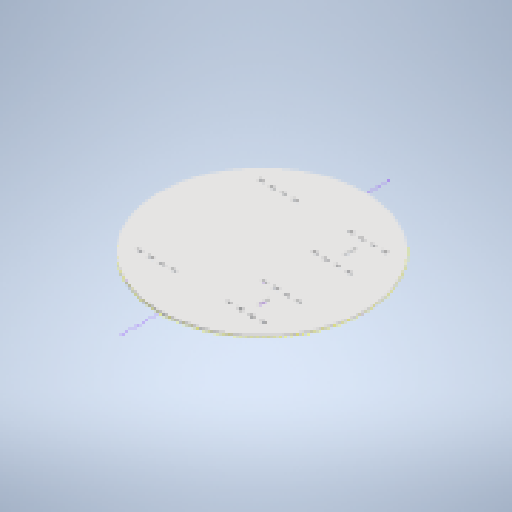
# Autodesk Inventor part: Osn. platform
Saved by Autodesk Inventor 2023.1 (Build 271208000, 208)
## iProperties
Created: 2023-03-13
Part Number: Osn. platform
Material: Типовые
Document SubType Name: Modeling
Designer: User
Density: 1 g/cm^3
Appearance: По умолчанию
Author: User
Autodesk Inventor part; units mm, degrees
ref_plane "YZ Plane" through (0, 0, 0) normal (1, 0, 0) x (0, 1, 0)
ref_plane "XZ Plane" through (0, 0, 0) normal (0, 1, 0) x (-1, 0, 0)
ref_plane "XY Plane" through (0, 0, 0) normal (0, 0, 1) x (1, 0, 0)
sketch "Основ. платформа" plane through (0, 0, 0) normal (0, 1, 0) x (-1, 0, 0)
  circle A0 centre (0, 0) radius 240
  dimension "d117" = 480
  constraints: 1 centre point, 1 coincident
  measures "d117" diameter of A0
extrude "Осн. платформа" add sketch "Основ. платформа" along normal blind 5
sketch "Эскиз14" plane through (0, 5, 0) normal (0, 1, 0) x (1, 0, 0)
  line L0 (137.6204, -61.9298) -> (150.9061, -61.9298) projected
  line L1 (150.9061, -61.9298) -> (150.9061, -55.9298) projected
  line L2 (137.6204, -55.9298) -> (150.9061, -55.9298) projected
  line L3 (137.6204, -61.9298) -> (137.6204, -55.9298) projected
  line L4 (111.049, -61.9298) -> (124.3347, -61.9298) projected
  line L5 (124.3347, -61.9298) -> (124.3347, -55.9298) projected
  line L6 (111.049, -55.9298) -> (124.3347, -55.9298) projected
  line L7 (111.049, -61.9298) -> (111.049, -55.9298) projected
  line L8 (84.4776, -61.9298) -> (97.7633, -61.9298) projected
  line L9 (97.7633, -61.9298) -> (97.7633, -55.9298) projected
  line L10 (84.4776, -55.9298) -> (97.7633, -55.9298) projected
  line L11 (84.4776, -61.9298) -> (84.4776, -55.9298) projected
  line L12 (57.9061, -144.9298) -> (71.1919, -144.9298) projected
  line L13 (71.1919, -144.9298) -> (71.1919, -138.9298) projected
  line L14 (57.9061, -138.9298) -> (71.1919, -138.9298) projected
  line L15 (57.9061, -144.9298) -> (57.9061, -138.9298) projected
  line L16 (84.4776, -144.9298) -> (97.7633, -144.9298) projected
  line L17 (97.7633, -144.9298) -> (97.7633, -138.9298) projected
  line L18 (84.4776, -138.9298) -> (97.7633, -138.9298) projected
  line L19 (84.4776, -144.9298) -> (84.4776, -138.9298) projected
  line L20 (111.049, -144.9298) -> (124.3347, -144.9298) projected
  line L21 (124.3347, -144.9298) -> (124.3347, -138.9298) projected
  line L22 (111.049, -138.9298) -> (124.3347, -138.9298) projected
  line L23 (111.049, -144.9298) -> (111.049, -138.9298) projected
  line L24 (137.6204, -144.9298) -> (150.9061, -144.9298) projected
  line L25 (150.9061, -144.9298) -> (150.9061, -138.9298) projected
  line L26 (137.6204, -138.9298) -> (150.9061, -138.9298) projected
  line L27 (137.6204, -144.9298) -> (137.6204, -138.9298) projected
  line L28 (101.4061, -87.5965) -> (101.4061, -113.2631) projected
  line L29 (101.4061, -113.2631) -> (107.4061, -113.2631) projected
  line L30 (107.4061, -113.2631) -> (107.4061, -87.5965) projected
  line L31 (107.4061, -87.5965) -> (101.4061, -87.5965) projected
  line L32 (57.9061, -61.9298) -> (71.1919, -61.9298) projected
  line L33 (71.1919, -61.9298) -> (71.1919, -55.9298) projected
  line L34 (57.9061, -55.9298) -> (71.1919, -55.9298) projected
  line L35 (57.9061, -61.9298) -> (57.9061, -55.9298) projected
  line L36 (-295.6598, 0) -> (443.256, 0) construction
  line L37 (0, -368.1913) -> (0, 462.3459) construction
  line L38 (-58.1024, -138.9298) -> (-70.9595, -138.9298) projected
  line L39 (-70.9595, -138.9298) -> (-70.9595, -144.9298) projected
  line L40 (-58.1024, -144.9298) -> (-70.9595, -144.9298) projected
  line L41 (-58.1024, -138.9298) -> (-58.1024, -144.9298) projected
  line L42 (-83.8167, -138.9298) -> (-96.6738, -138.9298) projected
  line L43 (-96.6738, -138.9298) -> (-96.6738, -144.9298) projected
  line L44 (-83.8167, -144.9298) -> (-96.6738, -144.9298) projected
  line L45 (-83.8167, -138.9298) -> (-83.8167, -144.9298) projected
  line L46 (-109.531, -138.9298) -> (-122.3881, -138.9298) projected
  line L47 (-122.3881, -138.9298) -> (-122.3881, -144.9298) projected
  line L48 (-109.531, -144.9298) -> (-122.3881, -144.9298) projected
  line L49 (-109.531, -138.9298) -> (-109.531, -144.9298) projected
  line L50 (-135.2452, -138.9298) -> (-148.1024, -138.9298) projected
  line L51 (-148.1024, -138.9298) -> (-148.1024, -144.9298) projected
  line L52 (-135.2452, -144.9298) -> (-148.1024, -144.9298) projected
  line L53 (-135.2452, -138.9298) -> (-135.2452, -144.9298) projected
  line L54 (-58.1024, -144.9298) -> (-148.1024, -144.9298) construction
  line L55 (-148.1024, -144.9298) -> (-148.1024, -100.7298) construction
  line L56 (-148.1024, -100.7298) -> (-58.1024, -100.7298) construction
  line L57 (-58.1024, -100.7298) -> (-58.1024, -144.9298) construction
  line L58 (-58.1024, -122.8298) -> (-148.1024, -122.8298) construction
  line L59 (137.6204, -138.9298) -> (124.3347, -144.9298) construction
  circle A0 centre (130.9776, -141.9298) radius 1.5
  circle A1 centre (104.2556, -141.9298) radius 1.5
  circle A2 centre (77.5336, -141.9298) radius 1.5
  circle A3 centre (130.9776, -58.9298) radius 1.5
  circle A4 centre (104.2556, -58.9298) radius 1.5
  circle A5 centre (77.5336, -58.9298) radius 1.5
  line L60 (-70.9595, -138.9298) -> (-83.8167, -144.9298) construction
  circle A6 centre (-77.3881, -141.9298) radius 1.5
  circle A7 centre (-103.2571, -141.9298) radius 1.5
  circle A8 centre (-129.1261, -141.9298) radius 1.5
  line L61 (-58.1024, -106.7298) -> (-70.9595, -106.7298)
  line L62 (-70.9595, -106.7298) -> (-70.9595, -100.7298)
  line L63 (-58.1024, -100.7298) -> (-70.9595, -100.7298)
  line L64 (-58.1024, -106.7298) -> (-58.1024, -100.7298)
  line L65 (-83.8167, -106.7298) -> (-96.6738, -106.7298)
  line L66 (-96.6738, -106.7298) -> (-96.6738, -100.7298)
  line L67 (-83.8167, -100.7298) -> (-96.6738, -100.7298)
  line L68 (-83.8167, -106.7298) -> (-83.8167, -100.7298)
  line L69 (-109.531, -106.7298) -> (-122.3881, -106.7298)
  line L70 (-122.3881, -106.7298) -> (-122.3881, -100.7298)
  line L71 (-109.531, -100.7298) -> (-122.3881, -100.7298)
  line L72 (-109.531, -106.7298) -> (-109.531, -100.7298)
  line L73 (-135.2452, -106.7298) -> (-148.1024, -106.7298)
  line L74 (-148.1024, -106.7298) -> (-148.1024, -100.7298)
  line L75 (-135.2452, -100.7298) -> (-148.1024, -100.7298)
  line L76 (-135.2452, -106.7298) -> (-135.2452, -100.7298)
  circle A9 centre (-77.3881, -103.7298) radius 1.5
  circle A10 centre (-103.2571, -103.7298) radius 1.5
  circle A11 centre (-129.1261, -103.7298) radius 1.5
  line L77 (137.6204, 61.9298) -> (150.9061, 61.9298)
  line L78 (150.9061, 61.9298) -> (150.9061, 55.9298)
  line L79 (137.6204, 55.9298) -> (150.9061, 55.9298)
  line L80 (137.6204, 61.9298) -> (137.6204, 55.9298)
  line L81 (111.049, 61.9298) -> (124.3347, 61.9298)
  line L82 (124.3347, 61.9298) -> (124.3347, 55.9298)
  line L83 (111.049, 55.9298) -> (124.3347, 55.9298)
  line L84 (111.049, 61.9298) -> (111.049, 55.9298)
  line L85 (84.4776, 61.9298) -> (97.7633, 61.9298)
  line L86 (97.7633, 61.9298) -> (97.7633, 55.9298)
  line L87 (84.4776, 55.9298) -> (97.7633, 55.9298)
  line L88 (84.4776, 61.9298) -> (84.4776, 55.9298)
  line L89 (57.9061, 144.9298) -> (71.1919, 144.9298)
  line L90 (71.1919, 144.9298) -> (71.1919, 138.9298)
  line L91 (57.9061, 138.9298) -> (71.1919, 138.9298)
  line L92 (57.9061, 144.9298) -> (57.9061, 138.9298)
  line L93 (84.4776, 144.9298) -> (97.7633, 144.9298)
  line L94 (97.7633, 144.9298) -> (97.7633, 138.9298)
  line L95 (84.4776, 138.9298) -> (97.7633, 138.9298)
  line L96 (84.4776, 144.9298) -> (84.4776, 138.9298)
  line L97 (111.049, 144.9298) -> (124.3347, 144.9298)
  line L98 (124.3347, 144.9298) -> (124.3347, 138.9298)
  line L99 (111.049, 138.9298) -> (124.3347, 138.9298)
  line L100 (111.049, 144.9298) -> (111.049, 138.9298)
  line L101 (137.6204, 144.9298) -> (150.9061, 144.9298)
  line L102 (150.9061, 144.9298) -> (150.9061, 138.9298)
  line L103 (137.6204, 138.9298) -> (150.9061, 138.9298)
  line L104 (137.6204, 144.9298) -> (137.6204, 138.9298)
  line L105 (101.4061, 87.5965) -> (101.4061, 113.2631)
  line L106 (101.4061, 113.2631) -> (107.4061, 113.2631)
  line L107 (107.4061, 113.2631) -> (107.4061, 87.5965)
  line L108 (107.4061, 87.5965) -> (101.4061, 87.5965)
  line L109 (57.9061, 61.9298) -> (71.1919, 61.9298)
  line L110 (71.1919, 61.9298) -> (71.1919, 55.9298)
  line L111 (57.9061, 55.9298) -> (71.1919, 55.9298)
  line L112 (57.9061, 61.9298) -> (57.9061, 55.9298)
  line L113 (0, 368.1913) -> (0, -462.3459) construction
  line L114 (-58.1024, 138.9298) -> (-70.9595, 138.9298)
  line L115 (-70.9595, 138.9298) -> (-70.9595, 144.9298)
  line L116 (-58.1024, 144.9298) -> (-70.9595, 144.9298)
  line L117 (-58.1024, 138.9298) -> (-58.1024, 144.9298)
  line L118 (-83.8167, 138.9298) -> (-96.6738, 138.9298)
  line L119 (-96.6738, 138.9298) -> (-96.6738, 144.9298)
  line L120 (-83.8167, 144.9298) -> (-96.6738, 144.9298)
  line L121 (-83.8167, 138.9298) -> (-83.8167, 144.9298)
  line L122 (-109.531, 138.9298) -> (-122.3881, 138.9298)
  line L123 (-122.3881, 138.9298) -> (-122.3881, 144.9298)
  line L124 (-109.531, 144.9298) -> (-122.3881, 144.9298)
  line L125 (-109.531, 138.9298) -> (-109.531, 144.9298)
  line L126 (-135.2452, 138.9298) -> (-148.1024, 138.9298)
  line L127 (-148.1024, 138.9298) -> (-148.1024, 144.9298)
  line L128 (-135.2452, 144.9298) -> (-148.1024, 144.9298)
  line L129 (-135.2452, 138.9298) -> (-135.2452, 144.9298)
  line L130 (-58.1024, 144.9298) -> (-148.1024, 144.9298) construction
  line L131 (-148.1024, 100.7298) -> (-58.1024, 100.7298) construction
  line L132 (137.6204, 138.9298) -> (124.3347, 144.9298) construction
  circle A12 centre (130.9776, 141.9298) radius 1.5
  circle A13 centre (104.2556, 141.9298) radius 1.5
  circle A14 centre (77.5336, 141.9298) radius 1.5
  circle A15 centre (130.9776, 58.9298) radius 1.5
  circle A16 centre (104.2556, 58.9298) radius 1.5
  circle A17 centre (77.5336, 58.9298) radius 1.5
  line L133 (-70.9595, 138.9298) -> (-83.8167, 144.9298) construction
  circle A18 centre (-77.3881, 141.9298) radius 1.5
  circle A19 centre (-103.2571, 141.9298) radius 1.5
  circle A20 centre (-129.1261, 141.9298) radius 1.5
  line L134 (-122.3881, 106.7298) -> (-122.3881, 100.7298)
  line L135 (-109.531, 100.7298) -> (-122.3881, 100.7298)
  line L136 (-109.531, 106.7298) -> (-109.531, 100.7298)
  line L137 (-109.531, 106.7298) -> (-122.3881, 106.7298)
  line L138 (-83.8167, 106.7298) -> (-96.6738, 106.7298)
  line L139 (-70.9595, 106.7298) -> (-70.9595, 100.7298)
  line L140 (-58.1024, 100.7298) -> (-70.9595, 100.7298)
  circle A21 centre (-103.2571, 103.7298) radius 1.5
  circle A22 centre (-129.1261, 103.7298) radius 1.5
  line L141 (-135.2452, 106.7298) -> (-135.2452, 100.7298)
  line L142 (-148.1024, 106.7298) -> (-148.1024, 100.7298)
  line L143 (-135.2452, 100.7298) -> (-148.1024, 100.7298)
  line L144 (-135.2452, 106.7298) -> (-148.1024, 106.7298)
  line L145 (-58.1024, 106.7298) -> (-70.9595, 106.7298)
  line L146 (-58.1024, 106.7298) -> (-58.1024, 100.7298)
  line L147 (-96.6738, 106.7298) -> (-96.6738, 100.7298)
  line L148 (-83.8167, 100.7298) -> (-96.6738, 100.7298)
  line L149 (-83.8167, 106.7298) -> (-83.8167, 100.7298)
  circle A23 centre (-77.3881, 103.7298) radius 1.5
  point P0 (0, 0)
  point P1 (-148.1024, -100.7298)
  point P2 (-58.1024, 122.8298)
  point P3 (-148.1024, 122.8298)
  point P4 (-148.1024, 100.7298)
  dimension "d129" = 90
  dimension "d130" = 44.2
  dimension "d131" = 3
  dimension "d134" = 26.722
  dimension "d137" = 83
  dimension "d140" = 3
  dimension "d143" = 25.869
  constraints: 196 end point, 106 symmetric about line, 24 centre point, 4 horizontal, 4 midpoint, 2 parallel, 2 vertical, 1 perpendicular, 29 other
  measures "d129" distance of L55.end L56.end
  measures "d130" distance of L54.end L55.end
  measures "d131" diameter of A0
  measures "d134" distance of A0.centre A1.centre
  measures "d137" distance of A0.centre A3.centre
  measures "d140" diameter of A6
  measures "d143" distance of A6.centre A7.centre
extrude "Выдавливание9" cut sketch "Эскиз14" against normal up to surface (5 mm away)
sketch "Эскиз13" plane through (0, 0, 0) normal (0, -1, 0) x (1, 0, 0)
  line L0 (0, 0) -> (172.9676, 166.3798) construction
  circle A0 centre (0, 0) radius 240 construction
  line L1 (0, 240) -> (240, 0) construction
  line L2 (104.4061, 0) -> (104.4061, 216.1003) construction
  line L3 (107.4061, 87.5961) -> (101.4061, 87.5961) construction
  line L4 (101.4061, 87.5961) -> (101.4061, 113.2631) construction
  line L5 (101.4061, 113.2631) -> (107.4061, 113.2631) construction
  line L6 (107.4061, 113.2631) -> (107.4061, 87.5961) construction
  line L7 (132.4776, 138.9298) -> (132.4776, 144.9298) construction
  line L8 (132.4776, 144.9298) -> (137.6204, 144.9298) construction
  line L9 (137.6204, 144.9298) -> (150.9061, 144.9298) construction
  line L10 (150.9061, 144.9298) -> (150.9061, 138.9298) construction
  line L11 (150.9061, 138.9298) -> (137.6204, 138.9298) construction
  line L12 (137.6204, 138.9298) -> (132.4776, 138.9298) construction
  line L13 (137.6204, 138.9298) -> (137.6204, 144.9298) construction
  line L14 (101.4061, 144.9298) -> (101.4061, 138.9298) construction
  line L15 (101.4061, 138.9298) -> (97.7633, 138.9298) construction
  line L16 (97.7633, 144.9298) -> (97.7633, 138.9298) construction
  line L17 (84.4776, 144.9298) -> (97.7633, 144.9298) construction
  line L18 (84.4776, 138.9298) -> (84.4776, 144.9298) construction
  line L19 (84.4776, 138.9298) -> (79.3347, 138.9298) construction
  line L20 (79.3347, 138.9298) -> (79.3347, 144.9298) construction
  line L21 (79.3347, 144.9298) -> (84.4776, 144.9298) construction
  line L22 (97.7633, 144.9298) -> (101.4061, 144.9298) construction
  line L23 (97.7633, 138.9298) -> (84.4776, 138.9298) construction
  line L24 (107.4061, 138.9298) -> (107.4061, 144.9298) construction
  line L25 (107.4061, 144.9298) -> (111.049, 144.9298) construction
  line L26 (111.049, 144.9298) -> (124.3347, 144.9298) construction
  line L27 (124.3347, 144.9298) -> (129.4776, 144.9298) construction
  line L28 (129.4776, 144.9298) -> (129.4776, 138.9298) construction
  line L29 (129.4776, 138.9298) -> (124.3347, 138.9298) construction
  line L30 (124.3347, 138.9298) -> (111.049, 138.9298) construction
  line L31 (111.049, 138.9298) -> (107.4061, 138.9298) construction
  line L32 (111.049, 138.9298) -> (111.049, 144.9298) construction
  line L33 (124.3347, 144.9298) -> (124.3347, 138.9298) construction
  line L34 (57.9061, 144.9298) -> (71.1919, 144.9298) construction
  line L35 (71.1919, 144.9298) -> (76.3347, 144.9298) construction
  line L36 (76.3347, 144.9298) -> (76.3347, 138.9298) construction
  line L37 (76.3347, 138.9298) -> (71.1919, 138.9298) construction
  line L38 (71.1919, 138.9298) -> (57.9061, 138.9298) construction
  line L39 (57.9061, 138.9298) -> (57.9061, 144.9298) construction
  line L40 (71.1919, 144.9298) -> (71.1919, 138.9298) construction
  circle A1 centre (0, 0) radius 240 construction
  line L41 (150.9061, -55.9298) -> (137.6204, -55.9298)
  line L42 (137.6204, -55.9298) -> (137.6204, -61.9298)
  line L43 (137.6204, -61.9298) -> (150.9061, -61.9298)
  line L44 (150.9061, -61.9298) -> (150.9061, -55.9298)
  line L45 (71.1919, -144.9298) -> (71.1919, -138.9298)
  line L46 (71.1919, -138.9298) -> (57.9061, -138.9298)
  line L47 (57.9061, -138.9298) -> (57.9061, -144.9298)
  line L48 (57.9061, -144.9298) -> (71.1919, -144.9298)
  line L49 (107.4061, 113.2631) -> (101.4061, 113.2631) construction
  line L50 (101.4061, 113.2631) -> (101.4061, 87.5965) construction
  line L51 (101.4061, 87.5965) -> (107.4061, 87.5965) construction
  line L52 (107.4061, 87.5965) -> (107.4061, 113.2631) construction
  line L53 (111.049, 144.9298) -> (111.049, 138.9298) construction
  line L54 (111.049, 138.9298) -> (124.3347, 138.9298) construction
  line L55 (124.3347, 138.9298) -> (124.3347, 144.9298) construction
  line L56 (124.3347, 144.9298) -> (111.049, 144.9298) construction
  line L57 (97.7633, 144.9298) -> (84.4776, 144.9298) construction
  line L58 (84.4776, 144.9298) -> (84.4776, 138.9298) construction
  line L59 (84.4776, 138.9298) -> (97.7633, 138.9298) construction
  line L60 (97.7633, 138.9298) -> (97.7633, 144.9298) construction
  line L61 (137.6204, -138.9298) -> (137.6204, -144.9298)
  line L62 (137.6204, -144.9298) -> (150.9061, -144.9298)
  line L63 (150.9061, -144.9298) -> (150.9061, -138.9298)
  line L64 (150.9061, -138.9298) -> (137.6204, -138.9298)
  line L65 (107.4061, -113.2631) -> (107.4061, -87.5965)
  line L66 (107.4061, -87.5965) -> (101.4061, -87.5965)
  line L67 (101.4061, -87.5965) -> (101.4061, -113.2631)
  line L68 (101.4061, -113.2631) -> (107.4061, -113.2631)
  line L69 (124.3347, -55.9298) -> (111.049, -55.9298)
  line L70 (111.049, -55.9298) -> (111.049, -61.9298)
  line L71 (111.049, -61.9298) -> (124.3347, -61.9298)
  line L72 (124.3347, -61.9298) -> (124.3347, -55.9298)
  line L73 (84.4776, -138.9298) -> (84.4776, -144.9298)
  line L74 (84.4776, -144.9298) -> (97.7633, -144.9298)
  line L75 (97.7633, -144.9298) -> (97.7633, -138.9298)
  line L76 (97.7633, -138.9298) -> (84.4776, -138.9298)
  line L77 (57.9061, -55.9298) -> (57.9061, -61.9298)
  line L78 (57.9061, -61.9298) -> (71.1919, -61.9298)
  line L79 (71.1919, -61.9298) -> (71.1919, -55.9298)
  line L80 (71.1919, -55.9298) -> (57.9061, -55.9298)
  line L81 (150.9061, 144.9298) -> (137.6204, 144.9298) construction
  line L82 (137.6204, 144.9298) -> (137.6204, 138.9298) construction
  line L83 (137.6204, 138.9298) -> (150.9061, 138.9298) construction
  line L84 (150.9061, 138.9298) -> (150.9061, 144.9298) construction
  line L85 (57.9061, 144.9298) -> (57.9061, 138.9298) construction
  line L86 (57.9061, 138.9298) -> (71.1919, 138.9298) construction
  line L87 (71.1919, 138.9298) -> (71.1919, 144.9298) construction
  line L88 (71.1919, 144.9298) -> (57.9061, 144.9298) construction
  line L89 (111.049, -144.9298) -> (124.3347, -144.9298)
  line L90 (124.3347, -144.9298) -> (124.3347, -138.9298)
  line L91 (124.3347, -138.9298) -> (111.049, -138.9298)
  line L92 (111.049, -138.9298) -> (111.049, -144.9298)
  line L93 (97.7633, -55.9298) -> (84.4776, -55.9298)
  line L94 (84.4776, -55.9298) -> (84.4776, -61.9298)
  line L95 (84.4776, -61.9298) -> (97.7633, -61.9298)
  line L96 (97.7633, -61.9298) -> (97.7633, -55.9298)
  line L97 (0, -35.6359) -> (0, 40.5263) construction
  line L98 (0, 0) -> (-172.9676, 166.3798) construction
  line L99 (0, 240) -> (-240, 0) construction
  line L100 (-104.4061, 0) -> (-104.4061, 216.1003) construction
  line L101 (-107.4061, 87.5961) -> (-101.4061, 87.5961) construction
  line L102 (-101.4061, 87.5961) -> (-101.4061, 113.2631) construction
  line L103 (-101.4061, 113.2631) -> (-107.4061, 113.2631) construction
  line L104 (-107.4061, 113.2631) -> (-107.4061, 87.5961) construction
  line L105 (-132.4776, 138.9298) -> (-132.4776, 144.9298) construction
  line L106 (-132.4776, 144.9298) -> (-137.6204, 144.9298) construction
  line L107 (-137.6204, 144.9298) -> (-150.9061, 144.9298) construction
  line L108 (-150.9061, 144.9298) -> (-150.9061, 138.9298) construction
  line L109 (-150.9061, 138.9298) -> (-137.6204, 138.9298) construction
  line L110 (-137.6204, 138.9298) -> (-132.4776, 138.9298) construction
  line L111 (-137.6204, 138.9298) -> (-137.6204, 144.9298) construction
  line L112 (-101.4061, 144.9298) -> (-101.4061, 138.9298) construction
  line L113 (-101.4061, 138.9298) -> (-97.7633, 138.9298) construction
  line L114 (-97.7633, 144.9298) -> (-97.7633, 138.9298) construction
  line L115 (-84.4776, 144.9298) -> (-97.7633, 144.9298) construction
  line L116 (-84.4776, 138.9298) -> (-84.4776, 144.9298) construction
  line L117 (-84.4776, 138.9298) -> (-79.3347, 138.9298) construction
  line L118 (-79.3347, 138.9298) -> (-79.3347, 144.9298) construction
  line L119 (-79.3347, 144.9298) -> (-84.4776, 144.9298) construction
  line L120 (-97.7633, 144.9298) -> (-101.4061, 144.9298) construction
  line L121 (-97.7633, 138.9298) -> (-84.4776, 138.9298) construction
  line L122 (-107.4061, 138.9298) -> (-107.4061, 144.9298) construction
  line L123 (-107.4061, 144.9298) -> (-111.049, 144.9298) construction
  line L124 (-111.049, 144.9298) -> (-124.3347, 144.9298) construction
  line L125 (-124.3347, 144.9298) -> (-129.4776, 144.9298) construction
  line L126 (-129.4776, 144.9298) -> (-129.4776, 138.9298) construction
  line L127 (-129.4776, 138.9298) -> (-124.3347, 138.9298) construction
  line L128 (-124.3347, 138.9298) -> (-111.049, 138.9298) construction
  line L129 (-111.049, 138.9298) -> (-107.4061, 138.9298) construction
  line L130 (-111.049, 138.9298) -> (-111.049, 144.9298) construction
  line L131 (-124.3347, 144.9298) -> (-124.3347, 138.9298) construction
  line L132 (-57.9061, 144.9298) -> (-71.1919, 144.9298) construction
  line L133 (-71.1919, 144.9298) -> (-76.3347, 144.9298) construction
  line L134 (-76.3347, 144.9298) -> (-76.3347, 138.9298) construction
  line L135 (-76.3347, 138.9298) -> (-71.1919, 138.9298) construction
  line L136 (-71.1919, 138.9298) -> (-57.9061, 138.9298) construction
  line L137 (-57.9061, 138.9298) -> (-57.9061, 144.9298) construction
  line L138 (-71.1919, 144.9298) -> (-71.1919, 138.9298) construction
  line L139 (-107.4061, 113.2631) -> (-101.4061, 113.2631) construction
  line L140 (-101.4061, 113.2631) -> (-101.4061, 87.5965) construction
  line L141 (-101.4061, 87.5965) -> (-107.4061, 87.5965) construction
  line L142 (-107.4061, 87.5965) -> (-107.4061, 113.2631) construction
  line L143 (-111.049, 144.9298) -> (-111.049, 138.9298) construction
  line L144 (-111.049, 138.9298) -> (-124.3347, 138.9298) construction
  line L145 (-124.3347, 138.9298) -> (-124.3347, 144.9298) construction
  line L146 (-124.3347, 144.9298) -> (-111.049, 144.9298) construction
  line L147 (-97.7633, 144.9298) -> (-84.4776, 144.9298) construction
  line L148 (-84.4776, 144.9298) -> (-84.4776, 138.9298) construction
  line L149 (-84.4776, 138.9298) -> (-97.7633, 138.9298) construction
  line L150 (-97.7633, 138.9298) -> (-97.7633, 144.9298) construction
  line L151 (-150.9061, 144.9298) -> (-137.6204, 144.9298) construction
  line L152 (-137.6204, 144.9298) -> (-137.6204, 138.9298) construction
  line L153 (-137.6204, 138.9298) -> (-150.9061, 138.9298) construction
  line L154 (-150.9061, 138.9298) -> (-150.9061, 144.9298) construction
  line L155 (-57.9061, 144.9298) -> (-57.9061, 138.9298) construction
  line L156 (-57.9061, 138.9298) -> (-71.1919, 138.9298) construction
  line L157 (-71.1919, 138.9298) -> (-71.1919, 144.9298) construction
  line L158 (-71.1919, 144.9298) -> (-57.9061, 144.9298) construction
  point P0 (104.4061, 100.4296)
  point P1 (-104.4061, 100.4296)
  dimension "d121" = 25.667
  constraints: 318 end point, 39 symmetric about line, 21 horizontal, 16 vertical, 4 point on circle, 2 parallel, 1 centre point, 1 perpendicular, 28 other
  measures "d121" distance of L3.end L4.end
